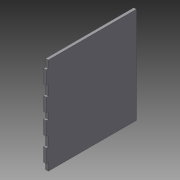
# Autodesk Inventor part: frount plate
Saved by Autodesk Inventor 2015 (Build 190159000, 159)
## iProperties
Created: 2014-07-26
Part Number: frount plate
Material: Generic
Document SubType Name: Modeling
Designer: karl
Density: 1 g/cm^3
Appearance: Default
Author: karl
Autodesk Inventor part; units mm, degrees
ref_plane "YZ Plane" through (0, 0, 0) normal (1, 0, 0) x (0, 1, 0)
ref_plane "XZ Plane" through (0, 0, 0) normal (0, 1, 0) x (-1, 0, 0)
ref_plane "XY Plane" through (0, 0, 0) normal (0, 0, 1) x (1, 0, 0)
sketch "Sketch1" plane through (0, 0, 0) normal (1, 0, 0) x (0, 1, 0)
  line L0 (-65, -71) -> (65, -71)
  line L1 (65, -71) -> (65, 71)
  line L2 (65, 71) -> (-65, 71)
  line L3 (-65, 71) -> (-65, -71)
  line L4 (-65, -71) -> (65, 71) construction
  line L5 (65, -71) -> (-65, 71) construction
  point P0 (0, 0)
  dimension "d0" = 130
  dimension "d1" = 142
  constraints: 12 end point, 2 midpoint, 2 parallel, 1 horizontal, 1 perpendicular
  measures "d0" distance of L2.end L1.end
  measures "d1" distance of L0.end L1.end
extrude "Extrusion1" add sketch "Sketch1" along normal blind 3
sketch "Sketch2" plane through (3, 0, 0) normal (1, 0, 0) x (0, 0, -1)
  line L0 (-71, -65) -> (71, -65) projected
  line L1 (-5, -65) -> (-25, -65)
  line L2 (-25, -65) -> (-25, -68)
  line L3 (-25, -68) -> (-5, -68)
  line L4 (-5, -68) -> (-5, -65)
  line L5 (-45, -65) -> (-65, -65)
  line L6 (-65, -65) -> (-65, -68)
  line L7 (-65, -68) -> (-45, -68)
  line L8 (-45, -68) -> (-45, -65)
  point P0 (0, 0)
  dimension "d4" = 20
  dimension "d5" = 3
  dimension "d6" = 5
  dimension "d7" = 20
  dimension "d8" = 3
  dimension "d9" = 20
  constraints: 16 end point, 4 parallel, 2 horizontal, 2 perpendicular, 2 point on line
  measures "d4" distance of L3.end L2.end
  measures "d5" distance of L2.end L1.end
  measures "d6" distance from line of L4 point (0, 0)
  measures "d7" distance of L7.end L6.end
  measures "d8" distance of L6.end L5.end
  measures "d9" distance between parallel lines of L2 L8
extrude "Extrusion2" add sketch "Sketch2" against normal blind 4
mirror "Mirror1" about plane through (0, 0, 0) normal (0, 0, 1) of "Extrusion2"
sketch "Sketch3" plane through (3, 0, 0) normal (1, 0, 0) x (0, 0, -1)
  line L0 (-60, -45) -> (-57, -45)
  line L1 (-57, -45) -> (-57, -60)
  line L2 (-57, -60) -> (-60, -60)
  line L3 (-60, -60) -> (-60, -45)
  line L4 (-71, -65) -> (-65, -65) projected
  point P0 (0, 0)
  dimension "d12" = 3
  dimension "d13" = 15
  dimension "d14" = 57
  dimension "d15" = 5
  constraints: 8 end point, 2 parallel, 1 horizontal, 1 perpendicular
  measures "d12" distance of L1.end L2.end
  measures "d13" distance of L0.end L1.end
  measures "d14" distance from line of point (0, 0) L1
  measures "d15" distance between parallel lines of L4 L2
extrude "Extrusion3" cut sketch "Sketch3" against normal blind 4
body "Solid1"
